Autodesk Fusion 360 part; units mm, degrees
(part 2 of 2)
sketch "Sketch1 (4)" plane through (0, 0, 154.45) normal (0, 0, 1) x (-1, 0, 0) in component "Top"
  circle A0 centre (0, 0) radius 32.5
  circle A1 centre (0, 0) radius 37.5
  circle A2 centre (0, 0) radius 31.5
  dimension "d41" = 65
  dimension "d42" = 75
  constraint concentric A0 A1
  measures "d41" diameter of A0
  measures "d42" diameter of A1
extrude "Extrude1''''" add sketch "Sketch1 (4)" against normal blind 12.7 separate body contours A1 makes body 5 in component "Top"
sketch "Sketch2 (3)" plane through (0, 0, 154.45) normal (0, 0, 1) x (-1, 0, 0) in component "Top"
  circle A0 centre (0, 0) radius 37.5
  circle A1 centre (0, 0) radius 37.5
  circle A2 centre (0, 0) radius 32.5
  dimension "d45" = 75
  measures "d45" diameter of A1
extrude "Extrude2'''" add sketch "Sketch2 (3)" along normal blind 6.35 contours A0 A1 | A2 bodies 5 in component "Top"
chamfer "Chamfer1'" distance 10 angle 45 1 edges at (34.9623, 13.5606, 160.8) on bodies 5 in component "Top"
chamfer "Chamfer2" distance 19 angle 45 1 edges at (19.5789, -7.5939, 25.4) on bodies 3 in component "Base"
sketch "Sketch5 (2)" plane through (0, 0, 154.45) normal (0, 0, 1) x (-1, 0, 0) in component "Shade"
  spline S0 degree 3 poles (23.6536, -15.6605) (25.8894, -12.6766) (27.5143, -9.2809) (29.4072, -1.9796) (29.6263, 1.8631) (28.583, 9.5024) (27.2995, 13.2206) (23.3503, 20.0368) (20.6956, 23.053) (15.3618, 27.161) (12.968, 28.5409) (7.8465, 30.6545) (5.1376, 31.3695) (2.3703, 31.7216) knots 0 0 0 0 1.118575 1.118575 2.261725 2.261725 3.42944 3.42944 4.621711 4.621711 5.44543 5.44543 6.280553 6.280553 6.280553 6.280553
  arc A0 (2.3703, 31.7216) -> (-22.9873, 21.9877) centre (0, 0) ccw
  spline S1 degree 3 poles (-22.9873, 21.9877) (-25.6611, 18.8847) (-27.7091, 15.2942) (-30.2729, 7.6039) (-30.7937, 3.5885) (-30.257, -4.3323) (-29.2362, -8.1631) (-25.8063, -15.1368) (-23.4587, -18.2259) (-18.662, -22.4692) (-16.5288, -23.9064) (-11.9724, -26.1609) (-9.5739, -26.9773) (-7.0991, -27.4654) knots 0 0 0 0 1.228802 1.228802 2.433005 2.433005 3.612599 3.612599 4.767575 4.767575 5.537325 5.537325 6.295652 6.295652 6.295652 6.295652
  arc A1 (-7.0991, -27.4654) -> (23.6536, -15.6605) centre (0, 0) ccw
  line L0 (-56, -42) -> (56, -42)
  line L1 (56, -42) -> (56, 42)
  line L2 (56, 42) -> (-56, 42)
  line L3 (-56, 42) -> (-56, -42)
  line L4 (-56, -42) -> (56, 42) construction
  line L5 (0, 0) -> (0, 0)
  constraint horizontal L0
  constraint perpendicular L0 L1
  constraint parallel L0 L2
  constraint parallel L1 L3
  constraint coincident L4 A0.centre
  constraint coincident L5 A0.centre
  constraint coincident A0.centre A1.centre
extrude "Extrude4'" [rolled back] along distance -65 taper angle 0 in component "Shade"
component "Plywood" placed x (1, 0, 0) y (0, 1, 0) z (0, 0, 1) at (0, 0, 0)
component "Bolt" placed x (1, 0, 0) y (0, 1, 0) z (0, 0, 1) at (0, 0, 0)
component "Base" placed x (1, 0, 0) y (0, 1, 0) z (0, 0, 1) at (0, 0, 0)
component "Shade" placed x (1, 0, 0) y (0, 1, 0) z (0, 0, 1) at (0, 0, 0)
component "Top" placed x (1, 0, 0) y (0, 1, 0) z (0, 0, 1) at (0, 0, 0)
equation "d9 = 2 in - 3 mm"
equation "d10 = 0.75 in - 4 mm"

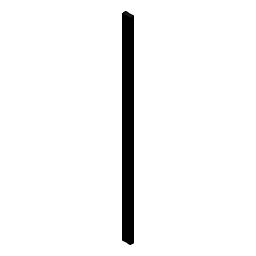
design "Rack Bar"
Autodesk Fusion 360 part; units mm, degrees
sketch "Sketch1" plane through (0, 0, 0) normal (0, 0, 1) x (1, 0, 0) in component "Rack"
  line L0 (266.7, 241.3) -> (-266.7, 241.3)
  line L1 (-266.7, 241.3) -> (-266.7, -241.3)
  line L2 (-266.7, -241.3) -> (266.7, -241.3)
  line L3 (266.7, -241.3) -> (266.7, 241.3)
  line L4 (266.7, 241.3) -> (-266.7, -241.3) construction
  line L5 (-266.7, 241.3) -> (266.7, -241.3) construction
  line L6 (266.7, -221.7638) -> (190.7, -221.7638)
  line L7 (190.7, -221.7638) -> (190.7, -253.2638)
  line L8 (190.7, -253.2638) -> (266.7, -253.2638)
  line L9 (266.7, -253.2638) -> (266.7, -221.7638)
  line L10 (266.7, 223.278) -> (190.7, 223.278)
  line L11 (190.7, 223.278) -> (190.7, 254.778)
  line L12 (190.7, 254.778) -> (266.7, 254.778)
  line L13 (266.7, 254.778) -> (266.7, 223.278)
  dimension "d22" = 533.4
  dimension "d23" = 482.6
  dimension "d99" = 76
  dimension "d100" = 31.5
  dimension "d101" = 76
  dimension "d102" = 31.5
  constraint perpendicular L0 L1
  constraint parallel L0 L2
  constraint parallel L1 L3
  constraint horizontal L0
  constraint coincident L4 origin
  constraint coincident L5 origin
  constraint horizontal L6
  constraint vertical L7
  constraint horizontal L8
  constraint vertical L9
  constraint coincident L3 L6.start
  constraint horizontal L10
  constraint vertical L11
  constraint horizontal L12
  constraint vertical L13
  constraint coincident L3 L10.start
  measures "d22" distance of L1.end L2.end
  measures "d23" distance of L0.end L1.end
  measures "d99" distance of L6.start L6.end
  measures "d100" distance of L6.start L8.end
  measures "d101" distance of L10.start L10.end
  measures "d102" distance of L10.start L12.end
extrude "Extrude1" add sketch "Sketch1" along normal blind 533.4 and the other way blind 1295.4 contours L2 L3 L6 L7 L9 | L2 L7 L8 L9 in component "Rack"
component "Rack" placed x (1, 0, 0) y (0, 1, 0) z (0, 0, 1) at (0, 0, 0)
equation "d103 = 6 ft - 21 in"
equation "d60 = ( 27.25 / 2 ) * 1 in - ( 23 / 2 ) * 1 in"
equation "d61 = ( 30 / 2 ) * 1 in - ( 27 / 2 ) * 1 in"
equation "d68 = ( 33.555 / 2 ) * 1 mm"
equation "d71 = ( 33.55 / 2 ) * 1 mm"
equation "d75 = ( 33.55 / 2 ) * 1 mm"
equation "d79 = ( 33.55 / 2 ) * 1 mm"
equation "d84 = ( 33.55 / 2 ) * 1 mm"
equation "d87 = ( 33.55 / 2 ) * 1 mm"
equation "d92 = ( 33.55 / 2 ) * 1 mm"
equation "d94 = ( 33.55 / 2 ) * 1 mm"

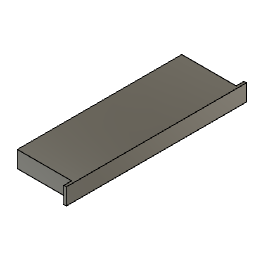
design "Power Unit"
Autodesk Fusion 360 part; units mm, degrees
sketch "Sketch1" plane through (0, 0, 0) normal (0, 0, 1) x (1, 0, 0)
  line L0 (76.2, 241.3) -> (-76.2, 241.3)
  line L1 (-76.2, 241.3) -> (-76.2, -241.3)
  line L2 (-76.2, -241.3) -> (76.2, -241.3)
  line L3 (76.2, -241.3) -> (76.2, 241.3)
  line L4 (76.2, 241.3) -> (-76.2, -241.3) construction
  line L5 (-76.2, 241.3) -> (76.2, -241.3) construction
  dimension "d1" = 152.4
  dimension "d2" = 482.6
  constraint perpendicular L0 L1
  constraint parallel L0 L2
  constraint parallel L1 L3
  constraint horizontal L0
  constraint coincident L4 origin
  constraint coincident L5 origin
  measures "d1" distance of L1.end L2.end
  measures "d2" distance of L0.end L1.end
extrude "Extrude1" add sketch "Sketch1" along normal blind 44.45
sketch "Sketch2" plane through (0, 0, 44.45) normal (0, 0, 1) x (-1, 0, 0)
  line L0 (-76.2, 241.3) -> (-76.2, -241.3)
  line L1 (-76.2, -241.3) -> (76.2, -241.3)
  line L2 (76.2, -241.3) -> (76.2, 241.3)
  line L3 (76.2, 241.3) -> (-76.2, 241.3)
  line L4 (-69.4, -241.3) -> (228.6, -241.3)
  line L5 (228.6, -241.3) -> (228.6, -220.3)
  line L6 (228.6, -220.3) -> (-69.4, -220.3)
  line L7 (-69.4, -220.3) -> (-69.4, -241.3)
  line L8 (-69.4, 241.3) -> (228.6, 241.3)
  line L9 (228.6, 241.3) -> (228.6, 220.3)
  line L10 (228.6, 220.3) -> (-69.4, 220.3)
  line L11 (-69.4, 220.3) -> (-69.4, 241.3)
  dimension "d5" = 21
  dimension "d6" = 21
  dimension "d7" = 298
  dimension "d8" = 298
  dimension "d11" = 6.8
  dimension "d12" = 6.8
  constraint horizontal L4
  constraint vertical L5
  constraint horizontal L6
  constraint vertical L7
  constraint coincident L1 L4.start
  constraint horizontal L8
  constraint vertical L9
  constraint horizontal L10
  constraint vertical L11
  constraint coincident L3 L8.start
  measures "d5" distance of L4.start L6.end
  measures "d6" distance of L8.start L10.end
  measures "d7" distance of L8.start L8.end
  measures "d8" distance of L5 L7
  measures "d11" distance of L0 L11
  measures "d12" distance of L0 L7
extrude "Extrude2" cut sketch "Sketch2" against normal up to surface (44.45 mm away) contours L2 L3 L8 L10 L11 | L1 L2 L4 L6 L7 | L2 L8 L9 L10 | L2 L4 L5 L6
equation "d11 = 1 ft - 298 mm"
equation "d12 = 1 ft - 298 mm"

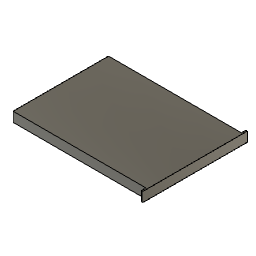
design "Super Pi Monitor"
Autodesk Fusion 360 part; units mm, degrees
sketch "Sketch1" plane through (0, 0, 0) normal (0, 0, 1) x (1, 0, 0)
  line L0 (310, 241.3) -> (-310, 241.3)
  line L1 (-310, 241.3) -> (-310, -241.3)
  line L2 (-310, -241.3) -> (310, -241.3)
  line L3 (310, -241.3) -> (310, 241.3)
  line L4 (310, 241.3) -> (-310, -241.3) construction
  line L5 (-310, 241.3) -> (310, -241.3) construction
  dimension "d1" = 620
  dimension "d2" = 482.6
  constraint perpendicular L0 L1
  constraint parallel L0 L2
  constraint parallel L1 L3
  constraint horizontal L0
  constraint coincident L4 origin
  constraint coincident L5 origin
  measures "d1" distance of L1.end L2.end
  measures "d2" distance of L0.end L1.end
extrude "Extrude1" add sketch "Sketch1" along normal blind 44.45
sketch "Sketch2" plane through (0, 0, 44.45) normal (0, 0, 1) x (-1, 0, 0)
  line L0 (-310, 241.3) -> (-310, -241.3)
  line L1 (-310, -241.3) -> (310, -241.3)
  line L2 (310, -241.3) -> (310, 241.3)
  line L3 (310, 241.3) -> (-310, 241.3)
  line L4 (-303.2, -241.3) -> (310, -241.3)
  line L5 (310, -241.3) -> (310, -220.3)
  line L6 (310, -220.3) -> (-303.2, -220.3)
  line L7 (-303.2, -220.3) -> (-303.2, -241.3)
  line L8 (-303.2, 241.3) -> (310, 241.3)
  line L9 (310, 241.3) -> (310, 220.3)
  line L10 (310, 220.3) -> (-303.2, 220.3)
  line L11 (-303.2, 220.3) -> (-303.2, 241.3)
  dimension "d5" = 21
  dimension "d6" = 21
  dimension "d11" = 6.8
  dimension "d12" = 6.8
  constraint horizontal L4
  constraint vertical L5
  constraint horizontal L6
  constraint vertical L7
  constraint coincident L1 L4.start
  constraint horizontal L8
  constraint vertical L9
  constraint horizontal L10
  constraint vertical L11
  constraint coincident L3 L8.start
  constraint collinear L2 L9
  constraint collinear L2 L5
  measures "d5" distance of L4.start L6.end
  measures "d6" distance of L8.start L10.end
  measures "d11" distance of L0 L11
  measures "d12" distance of L0 L7
extrude "Extrude2" cut sketch "Sketch2" against normal up to surface (44.45 mm away) contours L2 L3 L8 L9 L10 L11 | L1 L2 L4 L5 L6 L7
equation "d11 = 1 ft - 298 mm"
equation "d12 = 1 ft - 298 mm"

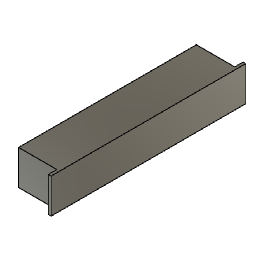
design "2U Space"
Autodesk Fusion 360 part; units mm, degrees
sketch "Sketch1" plane through (0, 0, 0) normal (0, 0, 1) x (1, 0, 0)
  line L0 (50.8, 241.3) -> (-50.8, 241.3)
  line L1 (-50.8, 241.3) -> (-50.8, -241.3)
  line L2 (-50.8, -241.3) -> (50.8, -241.3)
  line L3 (50.8, -241.3) -> (50.8, 241.3)
  line L4 (50.8, 241.3) -> (-50.8, -241.3) construction
  line L5 (-50.8, 241.3) -> (50.8, -241.3) construction
  dimension "d1" = 101.6
  dimension "d2" = 482.6
  constraint perpendicular L0 L1
  constraint parallel L0 L2
  constraint parallel L1 L3
  constraint horizontal L0
  constraint coincident L4 origin
  constraint coincident L5 origin
  measures "d1" distance of L1.end L2.end
  measures "d2" distance of L0.end L1.end
extrude "Extrude1" add sketch "Sketch1" along normal blind 86
sketch "Sketch2" plane through (0, 0, 86) normal (0, 0, 1) x (-1, 0, 0)
  line L0 (-50.8, 241.3) -> (-50.8, -241.3)
  line L1 (-50.8, -241.3) -> (50.8, -241.3)
  line L2 (50.8, -241.3) -> (50.8, 241.3)
  line L3 (50.8, 241.3) -> (-50.8, 241.3)
  line L4 (-44, -241.3) -> (254, -241.3)
  line L5 (254, -241.3) -> (254, -220.3)
  line L6 (254, -220.3) -> (-44, -220.3)
  line L7 (-44, -220.3) -> (-44, -241.3)
  line L8 (-44, 241.3) -> (254, 241.3)
  line L9 (254, 241.3) -> (254, 220.3)
  line L10 (254, 220.3) -> (-44, 220.3)
  line L11 (-44, 220.3) -> (-44, 241.3)
  dimension "d5" = 21
  dimension "d6" = 21
  dimension "d7" = 298
  dimension "d8" = 298
  dimension "d11" = 6.8
  dimension "d12" = 6.8
  constraint horizontal L4
  constraint vertical L5
  constraint horizontal L6
  constraint vertical L7
  constraint coincident L1 L4.start
  constraint horizontal L8
  constraint vertical L9
  constraint horizontal L10
  constraint vertical L11
  constraint coincident L3 L8.start
  measures "d5" distance of L4.start L6.end
  measures "d6" distance of L8.start L10.end
  measures "d7" distance of L8.start L8.end
  measures "d8" distance of L5 L7
  measures "d11" distance of L0 L11
  measures "d12" distance of L0 L7
extrude "Extrude2" cut sketch "Sketch2" against normal up to surface (86 mm away) contours L2 L3 L8 L10 L11 | L1 L2 L4 L6 L7 | L2 L8 L9 L10 | L2 L4 L5 L6
equation "d11 = 1 ft - 298 mm"
equation "d12 = 1 ft - 298 mm"
